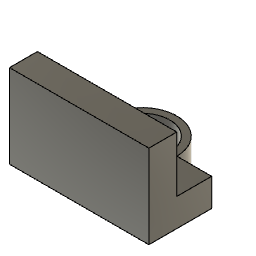
Model 8 (Autodesk Fusion 360 design; units mm, degrees)
Autodesk Fusion 360 part; units mm, degrees
sketch "Sketch1" plane through (0, 0, 0) normal (0, 0, 1) x (1, 0, 0)
  line L0 (0, 0) -> (100, 0)
  line L1 (100, 0) -> (100, 45)
  line L2 (100, 45) -> (0, 45)
  line L3 (0, 45) -> (0, 0)
  circle A0 centre (50, 45) radius 20
  arc A1 (75, 45) -> (25, 45) centre (50, 45) ccw
  dimension "d1" = 100
  dimension "d2" = 45
  dimension "d3" = 40
  dimension "d4" = 50
  constraint horizontal L0
  constraint vertical L1
  constraint horizontal L2
  constraint vertical L3
  constraint coincident L0.start L3.end
  constraint midpoint L2 A0.centre
  constraint concentric A0 A1
  constraint coincident L2 A1.end
  constraint coincident L2 A1.start
  measures "d1" distance of L0.start L0.end
  measures "d2" distance of L0.start L2.end
  measures "d3" diameter of A0
  measures "d4" diameter of A1
extrude "Extrude1" add sketch "Sketch1" along normal blind 20 contours L0 L1 L2 L3 A0 | L2 A0 A1
sketch "Sketch2" plane through (0, 0, 20) normal (0, 0, 1) x (-1, 0, 0)
  circle A0 centre (-50, -45) radius 20
  arc A1 (-75, -45) -> (-25, -45) centre (-50, -45) ccw
  line L0 (-25, -45) -> (0, -45)
  line L1 (0, -45) -> (0, 0)
  line L2 (0, 0) -> (-100, 0)
  line L3 (-100, 0) -> (-100, -45)
  line L4 (-100, -45) -> (-75, -45)
  line L5 (0, 0) -> (0, -20)
  line L6 (0, -20) -> (-100, -20)
  line L7 (-100, -20) -> (-100, 0)
  line L8 (-100, 0) -> (0, 0)
  dimension "d7" = 20
  constraint coincident L1.end L2.start
  constraint perpendicular L2 L5
  constraint coincident L3 L6.end
  constraint perpendicular L3 L6
  constraint coincident L2.end L3.start
  measures "d7" distance of L1.end L5.end
extrude "Extrude2" add sketch "Sketch2" along normal blind 40 contours L1 L2 L3 L5 L6 L7 L8
